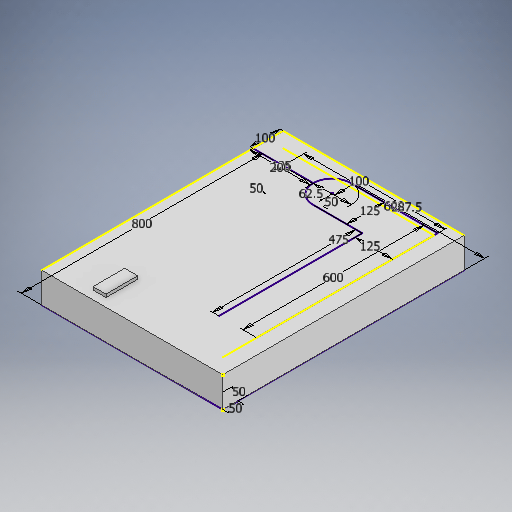
# Autodesk Inventor part: base
Saved by Autodesk Inventor 2025.3 (Build 293356000, 356)
## iProperties
Created: 2026-02-27
Part Number: base
Material: Generic
Document SubType Name: Modeling
Designer: user
Density: 1 g/cm^3
Appearance: Default
Author: user
Autodesk Inventor part; units mm, degrees
ref_plane "YZ Plane" through (0, 0, 0) normal (1, 0, 0) x (0, 1, 0)
sketch "Sketch1" plane through (0, 0, 0) normal (0, 1, 0) x (-1, 0, 0)
  line L0 (0, 0) -> (600, 0)
  line L1 (600, 0) -> (600, -800)
  line L2 (600, -800) -> (0, -800)
  line L3 (0, -800) -> (0, 0)
  line L4 (0, 0) -> (0, -50)
  line L5 (0, -50) -> (50, -50)
  line L6 (50, -50) -> (550, -50)
  line L7 (550, -50) -> (550, -750)
  line L8 (550, -750) -> (50, -750)
  line L9 (50, -750) -> (50, -50)
  dimension "d0" = 600
  dimension "d1" = 800
  dimension "d2" = 50
  dimension "d3" = 50
  dimension "d4" = 50
  dimension "d5" = 50
  constraints: 20 end point, 4 parallel, 3 perpendicular, 2 horizontal, 1 point on line
  measures "d0" distance of L1.end L2.end
  measures "d1" distance of L0.end L1.end
  measures "d2" distance of L0.start L4.end
  measures "d3" distance of L4.end L5.end
  measures "d4" distance between parallel lines of L2 L8
  measures "d5" distance between parallel lines of L1 L7
extrude "Extrusion1" add sketch "Sketch1" along normal blind 100 contours L6 L7 L8 L9 | L0 L1 L2 L3
extrude "Extrusion2" cut sketch "Sketch1" along normal blind 50 contours L6 L7 L8 L9
sketch "Sketch2" plane through (0, 100, 0) normal (0, 1, 0) x (1, 0, 0)
  line L0 (-600, 800) -> (-600, 0) projected
  line L1 (-600, 800) -> (-600, 700)
  line L2 (-600, 700) -> (-400, 700)
  arc A0 (-337.5, 762.5) -> (-337.5, 637.5) centre (-337.5, 700) ccw
  line L3 (-337.5, 762.5) -> (-50, 762.5)
  line L4 (-50, 750) -> (-550, 750) projected
  line L5 (-50, 762.5) -> (-50, 162.5)
  line L6 (-50, 50) -> (-50, 750) projected
  line L7 (-337.5, 637.5) -> (-175, 637.5)
  line L8 (-175, 637.5) -> (-175, 162.5)
  line L9 (0, 800) -> (-600, 800) projected
  point P0 (0, 0)
  dimension "d10" = 100
  dimension "d11" = 200
  dimension "d12" = 125
  dimension "d13" = 62.5
  dimension "d14" = 600
  dimension "d15" = 125
  dimension "d16" = 100
  dimension "d17" = 287.5
  dimension "d18" = 475
  dimension "d19" = 125
  constraints: 12 end point, 2 point on circle, 2 point on line, 1 centre point, 1 horizontal, 1 parallel, 1 perpendicular, 1 tangent, 1 vertical
  measures "d10" distance of L0.start L1.end
  measures "d11" distance of L1.end L2.end
  measures "d12" diameter of A0
  measures "d13" distance of L2.end A0.centre
  measures "d14" distance of L3.end L5.end
  measures "d15" distance from line of L5 L7.end
  measures "d16" distance from line of L9 A0.centre
  measures "d17" distance of L3.start L3.end
  measures "d18" distance of L7.end L8.end
  measures "d19" distance between parallel lines of L3 L7
ref_plane "Work Plane1" through (-600, 0, -150) normal (0, 0, 1) x (1, 0, 0)
sketch "Sketch5" plane through (0, 0, 0) normal (1, 0, 0) x (0, 0, -1)
  point P0 (0, 0)
ref_plane "Work Plane2" through (-150, 0, 0) normal (1, 0, 0) x (0, 0, -1)
sketch "Sketch10" plane through (0, 100, 0) normal (0, 1, 0) x (1, 0, 0)
  line L0 (-458, 28) -> (-415, 28)
  line L1 (-415, 28) -> (-415, 133)
  line L2 (-415, 133) -> (-458, 133)
  line L3 (-458, 133) -> (-458, 28)
  point P0 (0, 0)
  constraints: 8 end point, 2 parallel, 1 horizontal, 1 perpendicular
extrude "Extrusion9" add sketch "Sketch10" along normal blind 10
sketch "Sketch11" plane through (-415, 100, -133) normal (0, 0, -1) x (-1, 0, 0)
  circle A0 centre (21, 4) radius 0.5
  point P0 (-415, -100)
  dimension "d46" = 1
  constraints: 1 centre point
  measures "d46" diameter of A0
extrude "Extrusion10" cut sketch "Sketch11" against normal through all
body "Solid1"
